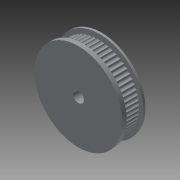
# Autodesk Inventor part: J1_DrivenPulley
Saved by Autodesk Inventor 2020 (Build 240168000, 168)
## iProperties
Created: 2015-06-17
Part Number: J1_DrivenPulley
Material: Generic
Document SubType Name: Modeling
Designer: Andrew
Density: 1 g/cm^3
Appearance: Default
Author: Andrew
Autodesk Inventor part; units mm, degrees
ref_plane "YZ Plane" through (0, 0, 0) normal (1, 0, 0) x (0, 1, 0)
ref_plane "XZ Plane" through (0, 0, 0) normal (0, 1, 0) x (-1, 0, 0)
ref_plane "XY Plane" through (0, 0, 0) normal (0, 0, 1) x (1, 0, 0)
sketch "Sketch1" plane through (0, 0, 0) normal (0, 0, 1) x (1, 0, 0)
  line L0 (0, 0) -> (0, 10.5) construction
  line L1 (0, 10.5) -> (2.5, 10.5) construction
  line L2 (2.5, 10.5) -> (19.8, 10.5)
  line L3 (19.8, 10.5) -> (19.8, 9.5)
  line L4 (19.8, 9.5) -> (18.3, 9.5)
  line L5 (18.3, 9.5) -> (18.3, 2)
  line L6 (18.3, 2) -> (19.8, 2)
  line L7 (19.8, 2) -> (19.8, 0)
  line L8 (19.8, 0) -> (2.5, 0)
  line L9 (2.5, 0) -> (2.5, 10.5)
  dimension "d0" = 2.5
  dimension "d1" = 7.5
  dimension "d2" = 2
  dimension "d4" = 1
  dimension "d6" = 18.3
  dimension "d15" = 1.5
  constraints: 20 end point, 5 perpendicular, 4 point on line, 1 horizontal, 1 parallel, 1 vertical
  measures "d0" distance between parallel lines of L0 L9
  measures "d1" distance of L4.end L5.end
  measures "d2" distance of L6.end L7.end
  measures "d4" distance between parallel lines of L2 L4
  measures "d6" distance between parallel lines of L0 L5
  measures "d15" distance between parallel lines of L3 L5
revolve "Revolution1" add sketch "Sketch1" angle 360 about axis through (0, 0, 0) along (0, 1, 0)
sketch "Sketch2" plane through (0, 2, 0) normal (0, 1, 0) x (1, 0, 0)
  line L0 (0, 0) -> (0, -18.3)
  circle A0 centre (0, -18.3) radius 1
  dimension "d8" = 2
  dimension "d9" = 18.3
  constraints: 2 end point, 1 centre point, 1 coincident, 1 vertical
  measures "d8" diameter of A0
  measures "d9" distance of L0.start L0.end
extrude "Extrusion1" cut sketch "Sketch2" along normal up to surface (7.5 mm away)
pattern_circular "Circular Pattern1" count 60 over 360 about axis through (0, 5.75, 0) along (0, -1, 0) of "Extrusion1"
body "Solid1"
